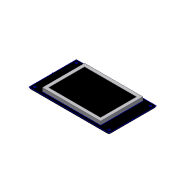
# Autodesk Inventor part: TFT Screen
Saved by Autodesk Inventor 2015 (Build 190159000, 159)
## iProperties
Created: 2018-04-21
Part Number: TFT Screen
Material: Generic
Document SubType Name: Modeling
Designer: Ghassan Yusuf
Density: 1 g/cm^3
Appearance: Default
Author: Ghassan Yusuf
Autodesk Inventor part; units mm, degrees
ref_plane "YZ Plane" through (0, 0, 0) normal (1, 0, 0) x (0, 1, 0)
ref_plane "XZ Plane" through (0, 0, 0) normal (0, 1, 0) x (-1, 0, 0)
ref_plane "XY Plane" through (0, 0, 0) normal (0, 0, 1) x (1, 0, 0)
sketch "TFT LCD Touch Screen" plane through (0, 0, 0) normal (0, 0, 1) x (1, 0, 0)
  line L0 (-40, 29) -> (40, 29)
  line L1 (40, 29) -> (40, -29)
  line L2 (40, -29) -> (-40, -29)
  line L3 (-40, -29) -> (-40, 29)
  line L4 (-55, 32.5) -> (55, 32.5)
  line L5 (55, 32.5) -> (55, -32.5)
  line L6 (55, -32.5) -> (-55, -32.5)
  line L7 (-55, -32.5) -> (-55, 32.5)
  circle A0 centre (-51, 28.5) radius 1.5
  circle A1 centre (-51, -28.5) radius 1.5
  circle A2 centre (51, -28.5) radius 1.5
  circle A3 centre (51, 28.5) radius 1.5
  point P0 (0.75, 3.075)
  point P1 (0, 29)
  point P2 (-40, 0)
  point P3 (0, 32.5)
  point P4 (55, 0)
  dimension "d0" = 110
  dimension "d1" = 65
  dimension "d2" = 3
  dimension "d3" = 57
  dimension "d4" = 102
  dimension "d5" = 4
  dimension "d6" = 4
  dimension "d7" = 80
  dimension "d8" = 58
  measures "d0" distance of L5.end L6.end
  measures "d1" distance of L4.end L5.end
  measures "d2" diameter of A0
  measures "d3" distance of A0.centre A1.centre
  measures "d4" distance of A3.centre A0.centre
  measures "d5" distance from line of L4 A3.centre
  measures "d6" distance from line of L7 A0.centre
  measures "d7" distance of L1.end L2.end
  measures "d8" distance of L0.end L1.end
sketch "Sketch1" plane through (0, 0, 0) normal (0, 0, 1) x (1, 0, 0)
  line L0 (-40, 29) -> (40, 29)
  line L1 (40, 29) -> (40, -29)
  line L2 (40, -29) -> (-40, -29)
  line L3 (-40, -29) -> (-40, 29)
  line L4 (-55, 32.5) -> (55, 32.5)
  line L5 (55, 32.5) -> (55, -32.5)
  line L6 (55, -32.5) -> (-55, -32.5)
  line L7 (-55, -32.5) -> (-55, 32.5)
  circle A0 centre (-51, 28.5) radius 1.5
  circle A1 centre (-51, -28.5) radius 1.5
  circle A2 centre (51, -28.5) radius 1.5
  circle A3 centre (51, 28.5) radius 1.5
  point P0 (0, 0)
  point P1 (-55, 0)
  constraints: 1 horizontal alignment, 3 other
extrude "Extrusion1" add sketch "Sketch1" against normal blind 1.5 contours L0 L1 L2 L3 | L4 L5 L6 L7
extrude "Extrusion2" add sketch "Sketch1" along normal blind 5 contours L0 L1 L2 L3
sketch "Sketch2" plane through (0, 0, 5) normal (0, 0, 1) x (1, 0, 0)
  line L0 (-40, 29) -> (40, 29)
  line L1 (40, 29) -> (40, -29)
  line L2 (40, -29) -> (-40, -29)
  line L3 (-40, -29) -> (-40, 29)
  line L4 (35.6625, 24.6625) -> (-35.6625, 24.6625)
  line L5 (-35.6625, 24.6625) -> (-35.6625, -24.6625)
  line L6 (-35.6625, -24.6625) -> (35.6625, -24.6625)
  line L7 (35.6625, -24.6625) -> (35.6625, 24.6625)
  point P0 (0, 0)
  constraints: 16 end point, 4 parallel, 2 perpendicular, 1 horizontal, 3 other
extrude "Extrusion3" cut sketch "Sketch2" against normal blind 0.2 contours L7 L6 L5 L4
fillet "Fillet1" radius 2 4 edges at (55, 32.5, -0.75) (-55, 32.5, -0.75) (-55, -32.5, -0.75) (55, -32.5, -0.75)
equation "\"d5\" = -0.5 * d3 + 0.5 * d1"
equation "\"d6\" = -0.5 * d4 + 0.5 * d0"
body "Solid1"
